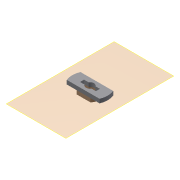
# Autodesk Inventor part: ECoG_holder_cap2
Saved by Autodesk Inventor 2014 (Build 180170000, 170)
## iProperties
Created: 2016-08-15
Part Number: ECoG_holder_cap2
Material: Generic
Document SubType Name: Modeling
Designer: Camilo
Density: 1 g/cm^3
Appearance: Default
Author: Camilo
Autodesk Inventor part; units mm, degrees
ref_plane "YZ Plane" through (0, 0, 0) normal (1, 0, 0) x (0, 1, 0)
ref_plane "XZ Plane" through (0, 0, 0) normal (0, 1, 0) x (-1, 0, 0)
ref_plane "XY Plane" through (0, 0, 0) normal (0, 0, 1) x (1, 0, 0)
ref_plane "Work Plane1" through (0, 0, 0) normal (0, 0, 1) x (1, 0, 0)
sketch "Sketch1" plane through (0, 0, 0) normal (0, 0, 1) x (1, 0, 0)
  arc A0 (-3.5454, 3.44) -> (-3.5454, -3.44) centre (0, 0) ccw construction
  line L0 (-3.5454, 3.44) -> (-1.1656, 3.44) construction
  line L1 (-1.1656, 3.44) -> (-1.1656, 4.44) construction
  line L2 (-1.1656, 4.44) -> (-2.5, 4.44) construction
  line L3 (-2.5, 4.44) -> (-2.5, 5.44) construction
  line L4 (-2.5, 5.44) -> (2.5, 5.44) construction
  line L5 (2.5, 5.44) -> (2.5, 4.44) construction
  line L6 (2.5, 4.44) -> (1.1656, 4.44) construction
  line L7 (1.1656, 4.44) -> (1.1656, 3.44) construction
  line L8 (1.1656, 3.44) -> (3.5454, 3.44) construction
  arc A1 (3.5454, -3.44) -> (3.5454, 3.44) centre (0, 0) ccw construction
  line L9 (1.1656, -3.44) -> (3.5454, -3.44) construction
  line L10 (1.1656, -4.44) -> (1.1656, -3.44) construction
  line L11 (1.1656, -4.44) -> (2.5, -4.44) construction
  line L12 (2.5, -4.44) -> (2.5, -5.44) construction
  line L13 (2.5, -5.44) -> (-2.5, -5.44) construction
  line L14 (-2.5, -5.44) -> (-2.5, -4.44) construction
  line L15 (-1.1656, -4.44) -> (-2.5, -4.44) construction
  line L16 (-1.1656, -3.44) -> (-1.1656, -4.44) construction
  line L17 (-3.5454, -3.44) -> (-1.1656, -3.44) construction
  arc A2 (-11, 8.1244) -> (-11, -8.1244) centre (0, 0) ccw projected
  line L18 (-11, -8.1244) -> (-11, -24.74) projected
  line L19 (-11, -24.74) -> (11, -24.74) projected
  line L20 (11, -24.74) -> (11, -8.1244) projected
  arc A3 (11, -8.1244) -> (11, 8.1244) centre (0, 0) ccw projected
  line L21 (11, 24.74) -> (11, 8.1244) projected
  line L22 (-11, 24.74) -> (11, 24.74) projected
  line L23 (-11, 8.1244) -> (-11, 24.74) projected
  line L24 (-8.2517, 3.44) -> (8.2517, 3.44)
  line L25 (8.2517, 3.44) -> (8.2517, -3.44)
  line L26 (8.2517, -3.44) -> (-8.2517, -3.44)
  line L27 (-8.2517, -3.44) -> (-8.2517, 3.44)
  arc A4 (8.2517, -3.44) -> (8.2517, 3.44) centre (0, 0) ccw
  arc A5 (-8.2517, 3.44) -> (-8.2517, -3.44) centre (0, 0) ccw
  point P0 (0, 0)
  constraints: 8 end point, 4 point on circle, 2 centre point, 1 coincident
extrude "Extrusion1" add sketch "Sketch1" along normal blind 2 contours L24 L25 L26 L27 | L27 A5 | A4 L25
sketch "Sketch2" plane through (0, 0, 0) normal (0, 0, -1) x (-1, 0, 0)
  line L0 (-8.2517, 3.44) -> (8.2517, 3.44) construction
  line L1 (8.2517, -3.44) -> (-8.2517, -3.44) construction
  line L2 (1.1656, -3.44) -> (3.5454, -3.44) construction
  line L3 (1.1656, -4.69) -> (1.1656, -3.44) construction
  line L4 (2.25, -4.69) -> (1.1656, -4.69) construction
  line L5 (2.25, -5.19) -> (2.25, -4.69) construction
  line L6 (-2.25, -5.19) -> (2.25, -5.19) construction
  line L7 (-2.25, -4.69) -> (-2.25, -5.19) construction
  line L8 (-1.1656, -4.69) -> (-2.25, -4.69) construction
  line L9 (-1.1656, -3.44) -> (-1.1656, -4.69) construction
  line L10 (-3.5454, -3.44) -> (-1.1656, -3.44) construction
  arc A0 (-3.5454, 3.44) -> (-3.5454, -3.44) centre (0, 0) ccw construction
  line L11 (-3.5454, 3.44) -> (-1.1656, 3.44) construction
  line L12 (-1.1656, 3.44) -> (-1.1656, 4.69) construction
  line L13 (-1.1656, 4.69) -> (-2.25, 4.69) construction
  line L14 (-2.25, 4.69) -> (-2.25, 5.19) construction
  line L15 (-2.25, 5.19) -> (2.25, 5.19) construction
  line L16 (2.25, 5.19) -> (2.25, 4.69) construction
  line L17 (2.25, 4.69) -> (1.1656, 4.69) construction
  line L18 (1.1656, 4.69) -> (1.1656, 3.44) construction
  line L19 (1.1656, 3.44) -> (3.5454, 3.44) construction
  arc A1 (3.5454, -3.44) -> (3.5454, 3.44) centre (0, 0) ccw construction
  circle A2 centre (0, 0) radius 6.94 construction
  circle A3 centre (0, 0) radius 4.79
  line L20 (-3.4814, 3.29) -> (3.4814, 3.29)
  line L21 (-3.4814, -3.29) -> (3.4814, -3.29)
  dimension "d3" = 0.15
  dimension "d4" = 0.15
  dimension "d5" = 0.15
  constraints: 4 end point, 4 point on circle, 2 horizontal, 1 centre point, 1 coincident
  measures "d3" radial gap between concentric circles of A0 A3
  measures "d4" distance between parallel lines of L20 L0
  measures "d5" distance between parallel lines of L21 L1
extrude "Extrusion2" add sketch "Sketch2" along normal blind 2 contours A3 L21 L20
sketch "Sketch3" plane through (0, 0, -2) normal (0, 0, -1) x (-1, 0, 0)
  arc A0 (3.4814, -3.29) -> (3.4814, 3.29) centre (0, 0) ccw projected
  circle A1 centre (0, 0) radius 2
  line L0 (-4, -1) -> (4, -1)
  line L1 (4, -1) -> (4, 1)
  line L2 (4, 1) -> (-4, 1)
  line L3 (-4, 1) -> (-4, -1)
  line L4 (-4, -1) -> (4, 1) construction
  line L5 (4, -1) -> (-4, 1) construction
  dimension "d8" = 4
  constraints: 12 end point, 2 midpoint, 1 centre point, 1 coincident
  measures "d8" diameter of A1
extrude "Extrusion3" cut sketch "Sketch3" against normal through all
body "Solid1"
